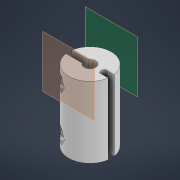
# Autodesk Inventor part: CouplerDIY2.0
Saved by Autodesk Inventor 2022 (Build 260153000, 153)
## iProperties
Created: 2023-11-11
Part Number: CouplerDIY2.0
Material: Všeobecné
Document SubType Name: Modeling
Designer: tada
Density: 1 g/cm^3
Appearance: Výchozí
Author: tada
Autodesk Inventor part; units mm, degrees
ref_plane "YZ Plane" through (0, 0, 0) normal (1, 0, 0) x (0, 1, 0)
ref_plane "XZ Plane" through (0, 0, 0) normal (0, 1, 0) x (-1, 0, 0)
ref_plane "XY Plane" through (0, 0, 0) normal (0, 0, 1) x (1, 0, 0)
sketch "Náčrt1" plane through (0, 0, 0) normal (0, 1, 0) x (-1, 0, 0)
  arc A0 (2.2226, 1.25) -> (2.2226, -1.25) centre (0, 0) ccw
  line L0 (8.9128, 1.25) -> (2.2226, 1.25)
  line L1 (2.2226, -1.25) -> (8.9128, -1.25)
  line L2 (7.3654, 0) -> (10.5772, 0) construction
  line L3 (-9.7024, 0) -> (-7.0449, 0) construction
  line L4 (-8.9128, 1.25) -> (-5.2128, 1.25)
  line L5 (-8.9128, -1.25) -> (-5.2128, -1.25)
  arc A1 (-5.2128, -1.25) -> (-5.2128, 1.25) centre (-6.774, 0) ccw
  arc A2 (8.9128, 1.25) -> (-8.9128, 1.25) centre (0, 0) ccw
  arc A3 (-8.9128, -1.25) -> (8.9128, -1.25) centre (0, 0) ccw
  line L6 (-2.05, 1.5166) -> (-2.05, -1.5166)
  arc A4 (2.2226, -1.25) -> (2.2226, 1.25) centre (0, 0) ccw construction
  dimension "d0" = 5.1
  dimension "d2" = 1.25
  dimension "d3" = 1.25
  dimension "d4" = 1.25
  dimension "d5" = 1.25
  dimension "d6" = 3.7
  dimension "d7" = 3.7
  dimension "d8" = 2
  dimension "d9" = 9
  dimension "d10" = 9
  dimension "d12" = 4.6
  constraints: 14 end point, 12 point on circle, 7 horizontal, 5 centre point, 2 coincident, 1 concentric, 1 parallel, 1 vertical
  measures "d0" diameter of A0
  measures "d2" distance between parallel lines of L2 L1
  measures "d3" distance between parallel lines of L0 L2
  measures "d4" distance between parallel lines of L4 L3
  measures "d5" distance between parallel lines of L5 L3
  measures "d6" distance of L4.start L4.end
  measures "d7" distance of L5.start L5.end
  measures "d8" radius of A1
  measures "d9" radius of A3
  measures "d10" radius of A2
extrude "Vysunutí1" add sketch "Náčrt1" along normal blind 30
sketch "Náčrt2" plane through (0, 30, 0) normal (0, 1, 0) x (1, 0, 0)
  point P0 (0, 0)
sketch "Náčrt3" plane through (0, 30, 0) normal (0, 1, 0) x (1, 0, 0)
  arc A0 (-2.078, -1.25) -> (-2.078, 1.25) centre (0, 0) ccw
  circle A1 centre (0, 0) radius 2.55
  line L0 (-2.2226, 1.25) -> (-1.532, 1.25)
  arc A2 (-2.2226, -1.25) -> (2.05, -1.5166) centre (0, 0) ccw projected
  line L1 (-2.2226, -1.25) -> (-1.6435, -1.25)
  dimension "d15" = 4.85
  dimension "d16" = 5.1
  constraints: 4 end point, 2 centre point, 2 coincident, 2 horizontal, 2 point on circle, 2 point on line
  measures "d15" diameter of A0
  measures "d16" diameter of A1
extrude "Vysunutí3" add sketch "Náčrt3" against normal blind 15 contours A0 L0 A1 L1 picked at (2.4543, 0)
extrude "Vysunutí4" cut sketch "Náčrt3" against normal blind 15 contours L1 A1 L0 A0 picked at (0.4889, -0.5637)
ref_plane "Pracovní rovina1" through (0, 30, -9) normal (0, 0, -1) x (-1, 0, 0)
ref_plane "Pracovní rovina2" through (0, 30, 9) normal (0, 0, 1) x (1, 0, 0)
sketch "Náčrt4" plane through (0, 30, -9) normal (0, 0, -1) x (-1, 0, 0)
  circle A0 centre (5.4128, -5.5) radius 2.9
  line L0 (8.9128, -30) -> (8.9128, 0) projected
  line L1 (8.9128, 0) -> (-8.9128, 0) projected
  circle A1 centre (5.4128, -5.5) radius 1.75
  circle A2 centre (5.4128, -24.5) radius 2.9
  circle A3 centre (5.4128, -24.5) radius 1.75
  line L2 (8.9128, -30) -> (-8.9128, -30) projected
  point P0 (0, -30)
  dimension "d23" = 3.5
  dimension "d24" = 5.5
  dimension "d25" = 5.8
  dimension "d26" = 3.5
  dimension "d27" = 3.5
  dimension "d28" = 5.8
  dimension "d29" = 3.5
  dimension "d30" = 5.5
  constraints: 4 centre point, 2 coincident
  measures "d23" distance from line of A0.centre L0
  measures "d24" distance from line of L1 A0.centre
  measures "d25" diameter of A0
  measures "d26" diameter of A1
  measures "d27" diameter of A3
  measures "d28" diameter of A2
  measures "d29" distance from line of L0 A2.centre
  measures "d30" distance from line of L2 A2.centre
extrude "Vysunutí5" cut sketch "Náčrt4" against normal blind 20 contours A1 | A3
extrude "Vysunutí6" cut sketch "Náčrt4" against normal blind 4
chamfer "Zkosení1" distance 0.5 angle 45 2 edges at (-3.6628, 24.5, -5) (-3.6628, 5.5, -5)
sketch "Náčrt5" plane through (0, 30, 9) normal (0, 0, 1) x (1, 0, 0)
  line L0 (-3.7673, -2.65) -> (-2.1219, -5.5)
  line L1 (-2.1219, -5.5) -> (-3.7673, -8.35)
  line L2 (-3.7673, -8.35) -> (-7.0582, -8.35)
  line L3 (-7.0582, -8.35) -> (-8.7037, -5.5)
  line L4 (-8.7037, -5.5) -> (-7.0582, -2.65)
  line L5 (-7.0582, -2.65) -> (-3.7673, -2.65)
  line L6 (8.9128, 0) -> (-8.9128, 0) projected
  line L7 (-8.9128, -30) -> (-8.9128, 0) projected
  arc A0 (-7.4833, -25.3805) -> (-7.4833, -23.6195) centre (-5.4128, -24.5) ccw projected
  line L8 (-7.0582, -21.65) -> (-3.7673, -21.65)
  line L9 (-3.7673, -21.65) -> (-2.1219, -24.5)
  line L10 (-2.1219, -24.5) -> (-3.7673, -27.35)
  line L11 (-3.7673, -27.35) -> (-7.0582, -27.35)
  line L12 (-7.0582, -27.35) -> (-8.7037, -24.5)
  line L13 (-8.7037, -24.5) -> (-7.0582, -21.65)
  line L14 (8.9128, -30) -> (-8.9128, -30) projected
  point P0 (0, -30)
  point P1 (-5.4128, -5.5)
  dimension "d38" = 5.7
  dimension "d39" = 5.5
  dimension "d40" = 3.5
  dimension "d41" = 5.5
  dimension "d42" = 5.7
  dimension "d43" = 5.5
  constraints: 24 end point, 1 coincident, 26 other
  measures "d38" distance between parallel lines of L0 L3
  measures "d39" distance from line of L6 point (-5.413, -5.5)
  measures "d40" distance from line of L7 point (-5.413, -5.5)
  measures "d41" distance from line of L6 L3.end
  measures "d42" distance between parallel lines of L12 L9
  measures "d43" distance from line of L14 L9.end
extrude "Vysunutí7" cut sketch "Náčrt5" against normal blind 4
equation "\"d3\" = d2"
equation "\"d5\" = d4"
equation "\"d7\" = d6"
equation "\"d27\" = d26"
equation "\"d28\" = d25"
equation "\"d29\" = d23"
equation "\"d30\" = d24"
equation "\"d42\" = d38"
